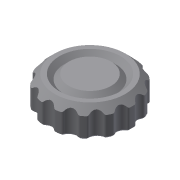
# Autodesk Inventor part: Knoob
Saved by Autodesk Inventor 2020 (Build 240168000, 168)
## iProperties
Created: 2022-10-11
Part Number: Knoob
Material: Allgemein
Document SubType Name: Modeling
Designer: uch10113
Density: 1 g/cm^3
Appearance: Vorgabe
Author: uch10113
Autodesk Inventor part; units mm, degrees
ref_plane "YZ Plane" through (0, 0, 0) normal (1, 0, 0) x (0, 1, 0)
ref_plane "XZ Plane" through (0, 0, 0) normal (0, 1, 0) x (-1, 0, 0)
ref_plane "XY Plane" through (0, 0, 0) normal (0, 0, 1) x (1, 0, 0)
sketch "Skizze1" plane through (0, 0, 0) normal (0, 0, 1) x (1, 0, 0)
  circle A0 centre (0, 0) radius 3
  circle A1 centre (0, 0) radius 9
  dimension "d0" = 6
  dimension "d1" = 18
  constraints: 2 centre point, 2 coincident
  measures "d0" diameter of A0
  measures "d1" diameter of A1
extrude "Extrusion1" add sketch "Skizze1" along normal blind 5
sketch "Skizze2" plane through (0, 0, 5) normal (0, 0, 1) x (1, 0, 0)
  circle A0 centre (0, 0) radius 9 projected
extrude "Extrusion2" add sketch "Skizze2" along normal blind 1
chamfer "Fase2" distance 1.5 angle 45 1 edges at (-9, 0, 6)
sketch "Skizze3" plane through (0, 0, 6) normal (0, 0, 1) x (1, 0, 0)
  circle A0 centre (0, 9.8251) radius 1.5484
  point P0 (0, 0)
  constraints: 1 centre point
extrude "Extrusion3" cut sketch "Skizze3" against normal blind 20
pattern_circular "Runde Anordnung1" count 14 over 360 about axis through (0, 0, 0) along (0, 0, 1) of "Extrusion3"
sketch "Skizze4" plane through (0, 0, 6) normal (0, 0, 1) x (1, 0, 0)
  circle A0 centre (0, 0) radius 7.5 projected
  circle A1 centre (0, 0) radius 6.5
  circle A2 centre (0, 0) radius 4.5
  dimension "d17" = 1
  dimension "d18" = 2
  constraints: 2 centre point
  measures "d17" radial gap between concentric circles of A0 A1
  measures "d18" radial gap between concentric circles of A1 A2
extrude "Extrusion4" cut sketch "Skizze4" against normal blind 1 contours A1
chamfer "Fase3" distance 1 angle 45 2 edges at (-6.5, 0, 5) (-4.5, 0, 5)
chamfer "Fase4" distance 1 angle 45 1 edges at (-3, 0, 0)
fillet "Rundung2" radius 0.5 2 edges at (-8.4108, 3.2029, 2.25) (-7.7482, 4.5789, 2.25)
pattern_circular "Runde Anordnung2" count 14 over 360 about axis through (0, 0, 0) along (0, 0, 1) of "Rundung2"
chamfer "Fase5" distance 0.5 angle 45 56 edges at (-9, 0, 0) (-8.919, -0.7058, 0) (-8.0692, -1.8417, 0) (-8.342, -3.234, 0) (-8.1087, -3.905, 0) (-7.7296, -4.5057, 0) (-6.471, -5.1604, 0) (-6.1127, -6.5331, 0) (-5.6114, -7.0365, 0) (-5.0091, -7.4132, 0) (-3.5911, -7.457, 0) (-2.6727, -8.5384, 0) (-2.0027, -8.7744, 0) (-1.2966, -8.8525, 0) (0, -8.2767, 0) (1.2966, -8.8525, 0) (2.0027, -8.7744, 0) (2.6727, -8.5384, 0) (3.5911, -7.457, 0) (5.0091, -7.4132, 0) (5.6114, -7.0365, 0) (6.1127, -6.5331, 0) (6.471, -5.1604, 0) (7.7296, -4.5057, 0) (8.1087, -3.905, 0) (8.342, -3.234, 0) (8.0692, -1.8417, 0) (8.919, -0.7058, 0) (9, 0, 0) (8.919, 0.7058, 0) (8.0692, 1.8417, 0) (8.342, 3.234, 0) (8.1087, 3.905, 0) (7.7296, 4.5057, 0) (6.471, 5.1604, 0) (6.1127, 6.5331, 0) (5.6114, 7.0365, 0) (5.0091, 7.4132, 0) (3.5911, 7.457, 0) (2.6727, 8.5384, 0) (2.0027, 8.7744, 0) (1.2966, 8.8525, 0) (0, 8.2767, 0) (-1.2966, 8.8525, 0) (-2.0027, 8.7744, 0) (-2.6727, 8.5384, 0) (-3.5911, 7.457, 0) (-5.0091, 7.4132, 0) (-5.6114, 7.0365, 0) (-6.1127, 6.5331, 0) (-6.471, 5.1604, 0) (-7.7296, 4.5057, 0) (-8.1087, 3.905, 0) (-8.342, 3.234, 0) (-8.0692, 1.8417, 0) (-8.919, 0.7058, 0)
sketch "Skizze5" plane through (0, 0, 0) normal (0, 0, -1) x (-1, 0, 0)
  circle A0 centre (0, 0) radius 3.15
  dimension "d35" = 6.3
  constraints: 1 centre point, 1 coincident
  measures "d35" diameter of A0
extrude "Extrusion5" cut sketch "Skizze5" against normal blind 5.5
